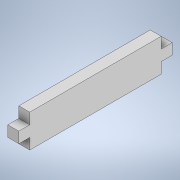
# Autodesk Inventor part: KabelBoxTest
Saved by Autodesk Inventor 2020.3 (Build 243373010, 373A)
## iProperties
Created: 2021-02-15
Part Number: KabelBoxTest
Material: Generisch
Document SubType Name: Modeling
Designer: Stefan
Density: 1 g/cm^3
Appearance: Vorgabe
Author: Stefan
Autodesk Inventor part; units mm, degrees
ref_plane "YZ Plane" through (0, 0, 0) normal (1, 0, 0) x (0, 1, 0)
ref_plane "XZ Plane" through (0, 0, 0) normal (0, 1, 0) x (-1, 0, 0)
ref_plane "XY Plane" through (0, 0, 0) normal (0, 0, 1) x (1, 0, 0)
sketch "Skizze4" plane through (0, 0, 0) normal (1, 0, 0) x (0, 1, 0)
  line L0 (-14.8108, -0.8671) -> (-14.8108, -120.8671)
  line L1 (15.1892, -120.8671) -> (15.1892, -0.8671)
  line L2 (5.1892, 9.1329) -> (-4.8108, 9.1329)
  line L3 (-4.8108, 9.1329) -> (-4.8108, -0.8671)
  line L4 (5.1892, -0.8671) -> (5.1892, 9.1329)
  line L5 (-4.8108, -120.8671) -> (-4.8108, -130.8671)
  line L6 (-4.8108, -130.8671) -> (5.1892, -130.8671)
  line L7 (5.1892, -130.8671) -> (5.1892, -120.8671)
  line L8 (15.1892, -0.8671) -> (5.1892, -0.8671)
  line L9 (-4.8108, -0.8671) -> (-14.8108, -0.8671)
  line L10 (-14.8108, -120.8671) -> (-4.8108, -120.8671)
  line L11 (5.1892, -120.8671) -> (15.1892, -120.8671)
  dimension "d8" = 30
  dimension "d9" = 120
  dimension "d10" = 10
  dimension "d11" = 10
  dimension "d12" = 10
  dimension "d13" = 10
  dimension "d16" = 10
  dimension "d17" = 10
  constraints: 24 end point, 7 parallel, 3 horizontal, 3 perpendicular
  measures "d8" distance of L1.start L0.end
  measures "d9" distance of L0.end L0.start
  measures "d10" distance of L4.start L3.end
  measures "d11" distance of L3.end L2.end
  measures "d12" distance of L6.end L5.end
  measures "d13" distance of L5.end L5.start
  measures "d16" distance between parallel lines of L1 L4
  measures "d17" distance between parallel lines of L1 L7
extrude "Extrusion3" add sketch "Skizze4" along normal blind 10
